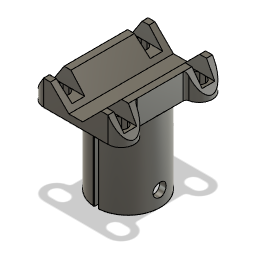
0.880.4094 - Demi-bride à embout - IGTE 21465_204506 (Autodesk Fusion 360 design; units mm, degrees)
Autodesk Fusion 360 part; units mm, degrees
sketch "Sketch1" plane through (0, 0, 0) normal (0, 0, 1) x (1, 0, 0)
  line L0 (0, 0) -> (0, 150) construction
  line L1 (-24.7, 0) -> (-24.7, 150) construction
  line L2 (-30.5, 0) -> (-30.5, 150) construction
  line L3 (0, 0) -> (-100, 0) construction
  line L4 (0, 60) -> (-100, 60) construction
  line L5 (-2, 0) -> (-2, 150) construction
  line L6 (0, 60) -> (0, 60)
  line L7 (-2, 58) -> (-2, 0)
  arc A0 (0, 60) -> (-2, 58) centre (0, 58) ccw
  line L8 (0, 101) -> (-100, 101) construction
  line L9 (0, 77) -> (-100, 77) construction
  line L10 (0, 85) -> (-100, 85) construction
  line L11 (0, 77) -> (100, 77) construction
  line L12 (-7.0711, 77) -> (-19.5787, 89.5076)
  line L13 (-30.5, 0) -> (-30.5, 101)
  line L14 (-30.5, 101) -> (-24, 101)
  line L15 (-24.7, 0) -> (-24.7, 87.3863)
  line L16 (-30.5, 0) -> (-24.7, 0)
  arc A1 (-19.5787, 89.5076) -> (-24.7, 87.3863) centre (-21.7, 87.3863) ccw
  line L17 (0, 77) -> (0, 83.5) construction
  line L18 (0, 83.5) -> (-6.5, 83.5)
  line L19 (-6.5, 83.5) -> (-24, 101)
  line L20 (0, 77) -> (-7.0711, 77)
  line L21 (0, 83.5) -> (0, 77)
  line L22 (-7.0711, 77) -> (-24.7, 77)
  dimension "d1" = 150
  dimension "d2" = 24.7
  dimension "d3" = 30.5
  dimension "d4" = 100
  dimension "d5" = 60
  dimension "d6" = 2
  dimension "d7" = 2
  dimension "d8" = 101
  dimension "d9" = 77
  dimension "d10" = 85
  dimension "d15" = 3
  dimension "d16" = 6.5
  constraint coincident L0.start L3.start
  constraint perpendicular L3 L7
  constraint tangent L7 A0
  constraint horizontal L11
  constraint coincident L8 L13.end
  constraint coincident L2 L13.end
  constraint perpendicular L8 L13
  constraint coincident L8 L14.end
  constraint perpendicular L1 L14
  constraint horizontal L8
  constraint perpendicular L10 L15
  constraint perpendicular L15 L16
  constraint tangent L12 A1
  constraint tangent L15 A1
  constraint perpendicular L5 L18
  constraint coincident L9 L12.start
  constraint perpendicular L5 L20
  constraint perpendicular L9 L21
  constraint coincident L1 L22.end
  constraint coincident L9 L22.end
  constraint coincident L15 L22.end
  measures "d1" distance of L0.start L0.end
  measures "d4" distance of L0.start L3.end
  measures "d7" radius of A0
  measures "d15" radius of A1
  measures "d16" distance of L9.start L17.end
revolve "Revolve1" add sketch "Sketch1" angle 360 about axis through (0, 1.75, 0) along (0, 1, 0)
sketch "Sketch2" plane through (0, 0, 0) normal (0, 0, 1) x (1, 0, 0)
  line L0 (24, 101) -> (-24, 101)
  line L1 (6.5, 83.5) -> (-6.5, 83.5)
  line L2 (24, 101) -> (6.5, 83.5)
  line L3 (-6.5, 83.5) -> (-24, 101)
  line L4 (-2, 58) -> (-2, 0)
  arc A0 (0, 60) -> (-2, 58) centre (0, 58) ccw
  line L5 (0, 101) -> (0, 0) construction
  line L6 (2, 58) -> (2, 0)
  arc A1 (2, 58) -> (0, 60) centre (0, 58) ccw
  line L7 (2, 0) -> (-2, 0)
  constraint coincident L0.start L2.start
  constraint coincident L1.start L2.end
  constraint coincident L1.end L3.start
  constraint coincident L0.end L3.end
  constraint midpoint L0 L5.start
  constraint coincident L5.end origin
  constraint symmetric L4.start L5 L6.start
  constraint symmetric L4.end L5 L6.end
  constraint symmetric A0.start L5 A1.end
  constraint symmetric A0 L5 A1
  constraint coincident L4.end L7.end
extrude "Extrude1" cut sketch "Sketch2" along normal through all and the other way through all
sketch "Sketch3" plane through (0, 0, 0) normal (1, 0, 0) x (0, 0, -1)
  line L0 (30.4344, 0) -> (-30.4344, 0) construction
  line L1 (30.4344, 15) -> (-30.4344, 15) construction
  line L2 (0, 15) -> (0, 0) construction
  circle A0 centre (0, 15) radius 6.25
  dimension "d20" = 15
  dimension "d21" = 12.5
  constraint midpoint L1 L2.start
  constraint coincident L2.end origin
  constraint perpendicular L0 L2
  constraint coincident L2.start A0.centre
  measures "d21" diameter of A0
extrude "Extrude2" cut sketch "Sketch3" along normal through all and the other way through all
fillet "Fillet1" radius 0.5 8 edges at (30.5, 0, 0) (-30.5, 0, 0) (2, 29, -30.4344) (0, 60, -30.5) (-2, 29, -30.4344) (-2, 29, 30.4344) (0, 60, 30.5) (2, 29, 30.4344)
sketch "Sketch de construction - Gabarit tube 38" plane through (0, 0, 0) normal (0, 0, 1) x (1, 0, 0)
  line L0 (-6.5, 83.5) -> (6.5, 83.5) construction
  line L1 (0, 0) -> (0, 83.5) construction
  line L2 (0, 83.5) -> (0, 103.8701) construction
  circle A0 centre (0, 103.8701) radius 19 construction
  line L3 (-24, 101) -> (-6.5, 83.5) construction
  line L4 (6.5, 83.5) -> (24, 101) construction
  line L5 (0, 103.8701) -> (-19, 103.8701) construction
  line L6 (0, 103.8701) -> (19, 103.8701) construction
  line L7 (19, 103.8701) -> (19, 96) construction
  line L8 (-19, 103.8701) -> (-19, 96) construction
  dimension "d25" = 38
  constraint coincident L1.start origin
  constraint midpoint L0 L1.end
  constraint perpendicular L0 L2
  constraint coincident L2.end A0.centre
  constraint tangent A0 L3
  constraint coincident A0 L5.end
  constraint perpendicular L2 L5
  constraint coincident A0 L6.end
  constraint perpendicular L2 L6
  constraint tangent A0 L7
  constraint tangent A0 L8
  constraint coincident L3 L8.end
  constraint coincident L4 L7.end
  measures "d25" diameter of A0
ref_plane "WorkPlane1" through (0, 101, 0) normal (0, 1, 0) x (0, 0, 1)
sketch "Sketch5" plane through (0, 101, 0) normal (0, 1, 0) x (1, 0, 0)
  line L0 (0, 0) -> (50, 0) construction
  line L1 (0, 0) -> (0, 50) construction
  line L2 (0, 0) -> (0, -50) construction
  line L3 (0, 0) -> (-50, 0) construction
  arc A0 (24, 18.8215) -> (6.5, 29.7993) centre (0, 0) ccw construction
  arc A1 (24, -18.8215) -> (24, 18.8215) centre (0, 0) ccw construction
  arc A2 (6.5, -29.7993) -> (24, -18.8215) centre (0, 0) ccw construction
  arc A3 (-6.5, -29.7993) -> (6.5, -29.7993) centre (0, 0) ccw construction
  arc A4 (-24, -18.8215) -> (-6.5, -29.7993) centre (0, 0) ccw construction
  arc A5 (-24, 18.8215) -> (-24, -18.8215) centre (0, 0) ccw construction
  arc A6 (-6.5, 29.7993) -> (-24, 18.8215) centre (0, 0) ccw construction
  arc A7 (6.5, 29.7993) -> (-6.5, 29.7993) centre (0, 0) ccw construction
  spline S0 degree 3 poles (-29.8528, -6.25) (-29.8665, -6.1869) (-29.8871, -6.0922) (-30.0102, -5.4537) (-30.097, -4.9731) (-30.2592, -3.8658) (-30.3452, -3.1645) (-30.4664, -1.6252) (-30.5, -0.7871) (-30.5, 0.7871) (-30.4664, 1.6252) (-30.3452, 3.1645) (-30.2592, 3.8658) (-30.097, 4.9731) (-30.0102, 5.4537) (-29.8871, 6.0922) (-29.8665, 6.1869) (-29.8583, 6.2248) knots 1.889202 1.889202 1.889202 1.889202 2.12536 2.12536 2.361518 2.361518 2.597661 2.597661 2.833804 2.833804 3.069947 3.069947 3.30609 3.30609 3.542247 3.542247 3.778405 3.778405 3.778405 3.778405 construction
  spline S1 degree 3 poles (29.8528, 6.25) (29.8665, 6.1869) (29.8871, 6.0922) (30.0102, 5.4537) (30.097, 4.9731) (30.2592, 3.8658) (30.3452, 3.1645) (30.4664, 1.6252) (30.5, 0.7871) (30.5, -0.7871) (30.4664, -1.6252) (30.3452, -3.1645) (30.2592, -3.8658) (30.097, -4.9731) (30.0102, -5.4537) (29.8871, -6.0922) (29.8665, -6.1869) (29.8596, -6.2184) knots 0 0 0 0 0.236158 0.236158 0.472315 0.472315 0.708458 0.708458 0.944601 0.944601 1.180744 1.180744 1.416887 1.416887 1.653045 1.653045 1.889202 1.889202 1.889202 1.889202 construction
  spline S2 degree 3 poles (-2.5417, 30.3939) (-2.5154, 30.3962) (-2.476, 30.3996) (-2.1382, 30.4257) (-1.754, 30.4533) (-0.8081, 30.4929) (-0.2542, 30.5036) (0.7318, 30.4945) (1.1676, 30.4798) (1.8074, 30.4477) (2.0418, 30.4321) (2.3449, 30.41) (2.4394, 30.4023) (2.525, 30.3953) (2.535, 30.3945) (2.5417, 30.3939) knots -0.785718 -0.785718 -0.785718 -0.785718 -0.687911 -0.687911 -0.524171 -0.524171 -0.365107 -0.365107 -0.231406 -0.231406 -0.128559 -0.128559 -0.049446 -0.049446 0 0 0 0 construction
  arc A8 (-2.5417, 30.3939) -> (-2.5417, -30.3939) centre (0, 0) ccw construction
  spline S3 degree 3 poles (2.5417, -30.3939) (2.5154, -30.3962) (2.476, -30.3996) (2.1382, -30.4257) (1.754, -30.4533) (0.8081, -30.4929) (0.2542, -30.5036) (-0.7318, -30.4945) (-1.1676, -30.4798) (-1.8074, -30.4477) (-2.0418, -30.4321) (-2.3449, -30.41) (-2.4394, -30.4023) (-2.525, -30.3953) (-2.535, -30.3945) (-2.5417, -30.3939) knots -0.785718 -0.785718 -0.785718 -0.785718 -0.687911 -0.687911 -0.524171 -0.524171 -0.365107 -0.365107 -0.231406 -0.231406 -0.128559 -0.128559 -0.049446 -0.049446 0 0 0 0 construction
  arc A9 (2.5417, -30.3939) -> (2.5417, 30.3939) centre (0, 0) ccw construction
  line L4 (6.5, -29.7993) -> (6.5, 29.7993) construction
  line L5 (-6.5, -29.7993) -> (-6.5, 29.7993) construction
  line L6 (-24, -18.8215) -> (-24, 18.8215) construction
  line L7 (24, 18.8215) -> (24, -18.8215) construction
  line L8 (0, 37) -> (-50, 37) construction
  line L9 (0, 37) -> (50, 37) construction
  line L10 (0, -37) -> (50, -37) construction
  line L11 (0, -37) -> (-50, -37) construction
  line L12 (-30.5, 0) -> (-30.5, -50) construction
  line L13 (-30.5, 0) -> (-30.5, 50) construction
  line L14 (30.5, 0) -> (30.5, 50) construction
  line L15 (30.5, 0) -> (30.5, -50) construction
  arc A10 (-30.5, 49.5) -> (-32.9194, 24.7364) centre (-30.5, 37) ccw
  line L16 (-30.5, 49.5) -> (0, 49.5)
  line L17 (-30.5, 0) -> (-30.5, 21.7931)
  arc A11 (-30.5, 21.7931) -> (-32.9194, 24.7364) centre (-33.5, 21.7931) ccw
  arc A12 (32.9194, 24.7364) -> (30.5, 49.5) centre (30.5, 37) ccw
  line L18 (30.5, 49.5) -> (0, 49.5)
  arc A13 (32.9194, 24.7364) -> (30.5, 21.7931) centre (33.5, 21.7931) ccw
  line L19 (30.5, 0) -> (30.5, 21.7931)
  arc A14 (-32.9194, -24.7364) -> (-30.5, -49.5) centre (-30.5, -37) ccw
  line L20 (-30.5, -49.5) -> (0, -49.5)
  arc A15 (30.5, -49.5) -> (32.9194, -24.7364) centre (30.5, -37) ccw
  arc A16 (-32.9194, -24.7364) -> (-30.5, -21.7931) centre (-33.5, -21.7931) ccw
  line L21 (-30.5, 0) -> (-30.5, -50) construction
  arc A17 (30.5, -21.7931) -> (32.9194, -24.7364) centre (33.5, -21.7931) ccw
  line L22 (30.5, 0) -> (30.5, -21.7931)
  line L23 (30.5, -49.5) -> (0, -49.5)
  line L24 (-19, 0) -> (-19, 75) construction
  line L25 (19, 0) -> (19, 75) construction
  line L26 (-19, 0) -> (-19, -75) construction
  line L27 (19, 0) -> (19, -75) construction
  circle A18 centre (-30.5, 37) radius 6 construction
  circle A19 centre (-25, 37) radius 6 construction
  line L28 (-30.5, 31) -> (-25, 31)
  line L29 (-30.5, 43) -> (-25, 43)
  arc A20 (-25, 31) -> (-25, 43) centre (-25, 37) ccw
  arc A21 (-30.5, 43) -> (-30.5, 31) centre (-30.5, 37) ccw
  line L30 (30.5, 31) -> (25, 31)
  arc A22 (30.5, 31) -> (30.5, 43) centre (30.5, 37) ccw
  line L31 (30.5, 43) -> (25, 43)
  arc A23 (25, 43) -> (25, 31) centre (25, 37) ccw
  arc A24 (-25, -43) -> (-25, -31) centre (-25, -37) ccw
  circle A25 centre (-25, -37) radius 6 construction
  line L32 (-30.5, -43) -> (-25, -43)
  arc A26 (-30.5, -31) -> (-30.5, -43) centre (-30.5, -37) ccw
  circle A27 centre (-30.5, -37) radius 6 construction
  line L33 (-30.5, -31) -> (-25, -31)
  arc A28 (30.5, -43) -> (30.5, -31) centre (30.5, -37) ccw
  line L34 (30.5, -43) -> (25, -43)
  arc A29 (25, -31) -> (25, -43) centre (25, -37) ccw
  line L35 (30.5, -31) -> (25, -31)
  line L36 (-30.5, -21.7931) -> (-30.5, 21.7931)
  circle A30 centre (0, 0) radius 30.5
  point P0 (-19, 0)
  point P1 (19, 0)
  dimension "d31" = 37
  dimension "d32" = 37
  dimension "d33" = 30.5
  dimension "d34" = 30.5
  dimension "d35" = 25
  dimension "d36" = 3
  dimension "d37" = 75
  dimension "d38" = 75
  dimension "d39" = 12
  dimension "d41" = 12
  constraint coincident L0.start L1.start
  constraint vertical L1
  constraint horizontal L0
  constraint vertical L2
  constraint horizontal L3
  constraint coincident L8 A10.centre
  constraint coincident L13 A10.centre
  constraint coincident L13 A10.start
  constraint tangent A10 L16
  constraint perpendicular L1 L16
  constraint coincident L1 L16.end
  constraint tangent A8 L17
  constraint tangent A10 A11
  constraint tangent L17 A11
  constraint symmetric L1 L12.start L14.start
  constraint symmetric L1 A10.start A12.end
  constraint symmetric L1 A10 A12
  constraint symmetric L1 L16.end L18.end
  constraint symmetric L1 L17.end A13.end
  constraint symmetric L1 A10.end A12.start
  constraint symmetric L1 A11 A13
  constraint symmetric L3 L12.start L13.start
  constraint symmetric L3 L13.end L12.end
  constraint symmetric L3 A10.start A14.end
  constraint symmetric L3 A10 A14
  constraint symmetric L3 L16.end L20.end
  constraint symmetric L3 L17.end A16.end
  constraint symmetric L3 A10.end A14.start
  constraint symmetric L3 A11 A16
  constraint symmetric L3 A12.end A15.start
  constraint symmetric L3 A12.start A15.end
  constraint symmetric L3 A12 A15
  constraint symmetric L3 A13.end A17.start
  constraint symmetric L3 A13 A17
  constraint symmetric L3 L14.start L15.start
  constraint coincident P0 L24.start
  constraint coincident P1 L25.start
  constraint symmetric L0 P0 L24.start
  constraint symmetric L0 L24.end L26.end
  constraint symmetric L0 P1 L25.start
  constraint symmetric L0 L25.end L27.end
  constraint concentric A10 A18
  constraint coincident A18 L28.start
  constraint coincident L13 L28.start
  constraint coincident A19 L28.end
  constraint tangent A19 L28
  constraint perpendicular L13 L28
  constraint coincident L13 L29.start
  constraint coincident A18 L29.start
  constraint coincident A19 L29.end
  constraint tangent A19 L29
  constraint perpendicular L13 L29
  constraint tangent L24 A20
  constraint symmetric L1 L28.start L30.start
  constraint symmetric L1 L28.end L30.end
  constraint symmetric L1 L29.start A22.end
  constraint symmetric L1 L29.end L31.end
  constraint symmetric L1 A20 A23
  constraint symmetric L1 A21 A22
  constraint symmetric L3 A18 A27
  constraint symmetric L3 A19 A25
  constraint symmetric L3 L28.start A26.start
  constraint symmetric L3 L28.end A24.end
  constraint symmetric L3 L29.start L32.start
  constraint symmetric L3 L29.end A24.start
  constraint symmetric L3 A20 A24
  constraint symmetric L3 A21 A26
  constraint symmetric L3 L30.start A28.end
  constraint symmetric L3 L30.end A29.start
  constraint symmetric L3 A22.end A28.start
  constraint symmetric L3 A22 A28
  constraint symmetric L3 L31.end L34.end
  constraint symmetric L3 A23 A29
  constraint tangent A11 L36
  measures "d35" diameter of A10
  measures "d36" radius of A11
  measures "d37" distance of P0 L24.end
  measures "d38" distance of P1 L25.end
  measures "d39" diameter of A18
  measures "d41" diameter of A19
extrude "Extrude3" add sketch "Sketch5" against normal blind 24 contours A10 L16 L17 A11 A12 L18 A13 L19 L36 A30 | A14 L20 A15 A16 A17 L22 L23 L36 A30
sketch "Sketch6" plane through (0, 0, 0) normal (0, 0, 1) x (1, 0, 0)
  line L0 (-6.5, 83.5) -> (6.5, 83.5)
  line L1 (-24, 101) -> (-6.5, 83.5)
  line L2 (6.5, 83.5) -> (24, 101)
  line L3 (30.5, 101) -> (30.5, 77) construction
  line L4 (30.5, 77) -> (30.5, 101) construction
  line L5 (43, 101) -> (30.5, 101) construction
  line L6 (32.9194, 101) -> (30.5, 101) construction
  line L7 (30.5, 77) -> (43, 77) construction
  line L8 (32.9194, 77) -> (30.5, 77) construction
  line L9 (-30.5, 101) -> (-32.9194, 101) construction
  line L10 (-30.5, 101) -> (-43, 101) construction
  line L11 (-43, 77) -> (-30.5, 77) construction
  line L12 (-30.5, 77) -> (-32.9194, 77) construction
  line L13 (36.5, 77) -> (30.5, 77) construction
  line L14 (30.5, 77) -> (25, 77) construction
  line L15 (25, 77) -> (19, 77) construction
  line L16 (25, 77) -> (30.5, 77) construction
  line L17 (-30.5, 77) -> (-36.5, 77) construction
  line L18 (-30.5, 77) -> (-25, 77) construction
  line L19 (-19, 77) -> (-25, 77) construction
  line L20 (-25, 77) -> (-30.5, 77) construction
  line L21 (30.5, 77) -> (43, 77) construction
  line L22 (32.9194, 77) -> (30.5, 77) construction
  line L23 (-30.5, 77) -> (30.5, 77) construction
  line L24 (-30.5, 77) -> (-32.9194, 77) construction
  line L25 (-43, 77) -> (-30.5, 77) construction
  line L26 (-30.5, 77) -> (30.5, 77) construction
  line L27 (24, 101) -> (-24, 101) construction
  line L28 (24, 101) -> (-24, 101) construction
  line L29 (-25, 101) -> (-30.5, 101) construction
  line L30 (-36.5, 101) -> (-30.5, 101) construction
  line L31 (-30.5, 101) -> (-25, 101) construction
  line L32 (-25, 101) -> (-19, 101) construction
  line L33 (30.5, 101) -> (36.5, 101) construction
  line L34 (30.5, 101) -> (25, 101) construction
  line L35 (19, 101) -> (25, 101) construction
  line L36 (25, 101) -> (30.5, 101) construction
  line L37 (30.5, 101) -> (36.5, 101) construction
  line L38 (30.5, 101) -> (25, 101) construction
  line L39 (19, 101) -> (25, 101) construction
  line L40 (25, 101) -> (30.5, 101) construction
  line L41 (-36.5, 101) -> (-30.5, 101) construction
  line L42 (-30.5, 101) -> (-25, 101) construction
  line L43 (-25, 101) -> (-19, 101) construction
  line L44 (-25, 101) -> (-30.5, 101) construction
  line L45 (32.9194, 101) -> (30.5, 101) construction
  line L46 (43, 101) -> (30.5, 101) construction
  line L47 (30.5, 101) -> (-30.5, 101) construction
  line L48 (-30.5, 101) -> (-43, 101) construction
  line L49 (-30.5, 101) -> (-32.9194, 101) construction
  line L50 (-30.5, 101) -> (-32.9194, 101) construction
  line L51 (-30.5, 101) -> (-43, 101) construction
  line L52 (-30.5, 101) -> (30.5, 101) construction
  line L53 (43, 101) -> (30.5, 101) construction
  line L54 (32.9194, 101) -> (30.5, 101) construction
  line L55 (-30.5, 101) -> (-30.5, 77) construction
  line L56 (-30.5, 77) -> (-30.5, 101) construction
  line L57 (-43, 101) -> (-43, 77) construction
  line L58 (43, 101) -> (43, 77) construction
  line L59 (43, 77) -> (43, 81) construction
  line L60 (43, 81) -> (30.5, 101)
  line L61 (43, 81) -> (43, 101)
  line L62 (43, 101) -> (30.5, 101)
  line L63 (-24, 101) -> (24, 101)
  line L64 (-43, 77) -> (-43, 81) construction
  line L65 (-43, 81) -> (-30.5, 101)
  line L66 (-30.5, 101) -> (-43, 101)
  line L67 (-43, 81) -> (-43, 101)
  point P0 (30.5, 101)
  point P1 (-30.5, 101)
  point P2 (-30.5, 77)
  dimension "d44" = 4
  dimension "d45" = 4
  constraint coincident L10.end L48.end
  constraint coincident L11.start L25.start
  constraint coincident L5.start L46.start
  constraint coincident L7.end L21.end
  constraint coincident P0 L3.start
  constraint perpendicular L5 L61
  constraint coincident L1.start L27.end
  constraint coincident L2.end L27.start
  constraint coincident P1 L9.start
  constraint perpendicular L10 L67
  measures "d44" distance of L7.end L59.end
  measures "d45" distance of L11.start L64.end
extrude "Extrude4" cut sketch "Sketch6" along normal through all and the other way through all
sketch "Sketch7" plane through (0, 0, 0) normal (1, 0, 0) x (0, 0, -1)
  arc A0 (-42.9161, 101) -> (-31.0839, 101) centre (-37, 102) ccw construction
  ellipse E0 centre (-37, 101) end of major axis (-37, 110.6) minor radius 6 (-43, 101) -> (-31, 101) ccw construction
  ellipse E1 centre (-37, 101) end of major axis (-37, 81) minor radius 12.5 (-49.5, 101) -> (-24.7364, 97.129) ccw construction
  line L0 (-37, 102) -> (-37, 81) construction
  line L1 (0, 0) -> (0, 83.5)
  line L2 (0, 0) -> (0, 83.5) construction
  line L3 (-37, 102) -> (-44, 102)
  line L4 (-37, 102) -> (-30, 102)
  line L5 (-37, 102) -> (-37, 87)
  line L6 (-37, 87) -> (-43, 87)
  line L7 (-43, 87) -> (-44, 102)
  line L8 (-31, 87) -> (-30, 102)
  line L9 (-37, 87) -> (-31, 87)
  line L10 (37, 87) -> (43, 87)
  line L11 (37, 87) -> (31, 87)
  line L12 (31, 87) -> (30, 102)
  line L13 (43, 87) -> (44, 102)
  line L14 (37, 102) -> (44, 102)
  line L15 (37, 102) -> (30, 102)
  point P0 (0, 83.5)
  dimension "d48" = 7
  dimension "d49" = 7
  dimension "d50" = 15
  dimension "d51" = 6
  constraint coincident A0.centre L0.start
  constraint coincident E1 L0.end
  constraint vertical L0
  constraint coincident L1.start L2.start
  constraint coincident P0 L1.end
  constraint symmetric L0 L3.end L4.end
  constraint symmetric L0 L5.end L6.start
  constraint symmetric L0 L6.end L8.start
  constraint symmetric A0.centre L2 L14.start
  constraint symmetric L2 L3.end L13.end
  constraint symmetric L2 L4.end L12.end
  constraint symmetric L2 L5.end L10.start
  constraint symmetric L2 L6.end L10.end
  constraint symmetric L2 L8.start L11.end
  measures "d48" distance of A0.centre L3.end
  measures "d49" distance of A0.centre L4.end
  measures "d50" distance of A0.centre L5.end
  measures "d51" distance of L5.end L6.end
extrude "Extrude5" cut sketch "Sketch7" along normal through all and the other way through all
